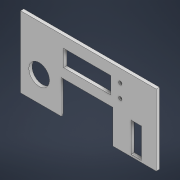
# Autodesk Inventor part: gora pudla
Saved by Autodesk Inventor 2022 (Build 260153000, 153)
## iProperties
Created: 2023-03-26
Part Number: gora pudla
Material: Generic
Document SubType Name: Modeling
Designer: patryk-komputer
Density: 1 g/cm^3
Appearance: Default
Author: patryk-komputer
Autodesk Inventor part; units mm, degrees
ref_plane "YZ Plane" through (0, 0, 0) normal (1, 0, 0) x (0, 1, 0)
ref_plane "XZ Plane" through (0, 0, 0) normal (0, 1, 0) x (-1, 0, 0)
ref_plane "XY Plane" through (0, 0, 0) normal (0, 0, 1) x (1, 0, 0)
sketch "Sketch1" plane through (0, 0, 0) normal (0, 0, 1) x (1, 0, 0)
  line L0 (0, 0) -> (210, 0)
  line L1 (210, 0) -> (210, 110)
  line L2 (210, 110) -> (0, 110)
  line L3 (0, 110) -> (0, 0)
  line L4 (66.5, 93) -> (139.5, 93)
  line L5 (139.5, 93) -> (139.5, 67)
  line L6 (139.5, 67) -> (66.5, 67)
  line L7 (66.5, 67) -> (66.5, 93)
  line L8 (63, 0) -> (63, 50)
  line L9 (63, 50) -> (143, 50)
  line L10 (143, 50) -> (143, 0)
  line L11 (63, 50) -> (63, 110) construction
  circle A0 centre (28.854, 39) radius 16
  line L12 (139.5, 93) -> (144.5, 93)
  line L13 (144.5, 93) -> (144.5, 67)
  line L14 (144.5, 67) -> (139.5, 67)
  circle A1 centre (154.5, 90.4) radius 2.6
  circle A2 centre (154.5, 69.6) radius 2.6
  line L15 (171, 13) -> (187, 13) construction
  line L16 (171, 44) -> (187, 44) construction
  line L17 (171, 49) -> (187, 49)
  line L18 (187, 49) -> (187, 3)
  line L19 (187, 3) -> (171, 3)
  line L20 (171, 3) -> (171, 49)
  line L21 (179, 49) -> (179, 3) construction
  line L22 (63, 50) -> (61, 50)
  line L23 (61, 50) -> (61, 0)
  line L24 (143, 50) -> (145, 50)
  line L25 (145, 50) -> (145, 0)
  line L26 (63, 50) -> (63, 52)
  line L27 (143, 50) -> (143, 52)
  line L28 (143, 52) -> (63, 52)
  point P0 (103, 93)
  point P1 (105, 110)
  point P2 (66.5, 80)
  point P3 (63, 80)
  point P4 (103, 50)
  dimension "d0" = 210
  dimension "d1" = 110
  dimension "d2" = 73
  dimension "d3" = 26
  dimension "d4" = 50
  dimension "d5" = 80
  dimension "d6" = 32
  dimension "d7" = 28.854
  dimension "d8" = 39
  dimension "d9" = 63
  dimension "d11" = 5
  dimension "d12" = 5.2
  dimension "d13" = 10
  dimension "d17" = 13
  dimension "d18" = 44
  dimension "d19" = 5
  dimension "d20" = 10
  dimension "d21" = 16
  dimension "d22" = 31
  dimension "d27" = 2
  constraints: 58 end point, 12 perpendicular, 10 point on line, 7 horizontal, 7 midpoint, 6 parallel, 3 centre point, 2 equal length, 2 tangent, 2 vertical, 2 vertical alignment, 1 equal radius, 1 horizontal alignment
  measures "d0" distance of L2.end L1.end
  measures "d1" distance of L1.end L0.end
  measures "d2" distance of L5.end L6.end
  measures "d3" distance of L4.end L5.end
  measures "d4" distance between parallel lines of L0 L9
  measures "d5" distance of L8.end L9.end
  measures "d6" diameter of A0
  measures "d7" distance from line of L3 A0.centre
  measures "d8" distance from line of L0 A0.centre
  measures "d9" distance between parallel lines of L3 L8
  measures "d11" distance between parallel lines of L5 L13
  measures "d12" diameter of A1
  measures "d13" distance from line of L13 A2.centre
  measures "d17" distance between parallel lines of L0 L15
  measures "d18" distance between parallel lines of L0 L16
  measures "d19" distance between parallel lines of L17 L16
  measures "d20" distance between parallel lines of L19 L15
  measures "d21" distance between parallel lines of L18 L20
  measures "d22" distance between parallel lines of L1 L21
  measures "d27" distance of L8.end L22.end
extrude "Extrusion1" add sketch "Sketch1" against normal blind 5 contours L3 L2 L1 L0 L25 L24 L27 L28 L26 L22 L23 | L26 L28 L27 L9
extrude "Extrusion2" add sketch "Sketch1" against normal blind 2 contours L12 L13 L14 L5
extrude "Extrusion3" add sketch "Sketch1" against normal blind 2 contours L23 L22 L8 L0 | L10 L24 L25 L0
extrude "Extrusion4" cut sketch "Sketch1" against normal blind 2 contours L26 L28 L27 L9
body "Solid1"
